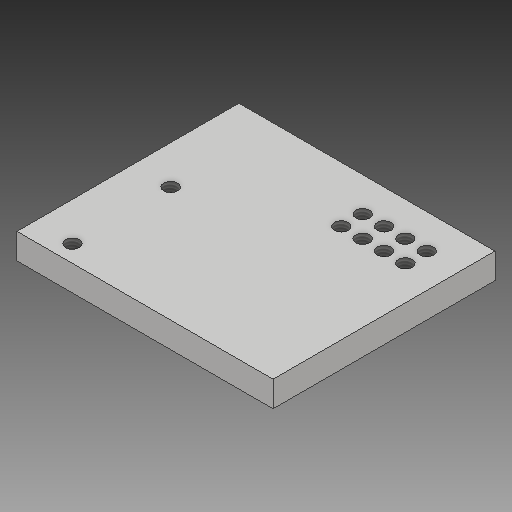
# Autodesk Inventor part: 160624 base pequeña laser
Saved by Autodesk Inventor 2019.2 (Build 232265000, 265)
## iProperties
Created: 2016-06-28
Part Number: 160624 base pequeña laser
Material: Generic
Document SubType Name: Modeling
Designer: Luis Villegas
Density: 1 g/cm^3
Appearance: Default
Author: Luis Villegas
Autodesk Inventor part; units mm, degrees
ref_plane "YZ Plane" through (0, 0, 0) normal (1, 0, 0) x (0, 1, 0)
ref_plane "XZ Plane" through (0, 0, 0) normal (0, 1, 0) x (-1, 0, 0)
ref_plane "XY Plane" through (0, 0, 0) normal (0, 0, 1) x (1, 0, 0)
sketch "Sketch1" plane through (0, 0, 0) normal (0, 1, 0) x (-1, 0, 0)
  line L0 (0, 0) -> (-52, 0)
  line L1 (-52, 0) -> (-52, -60)
  line L2 (-52, -60) -> (0, -60)
  line L3 (0, -60) -> (0, 0)
  dimension "d0" = 52
  dimension "d1" = 60
  constraints: 8 end point, 2 parallel, 1 coincident, 1 horizontal, 1 perpendicular
  measures "d0" distance of L2.end L1.end
  measures "d1" distance of L1.end L0.end
extrude "Extrusion1" add sketch "Sketch1" against normal blind 6
sketch "Sketch2" plane through (0, 0, 0) normal (0, 1, 0) x (1, 0, 0)
  line L0 (0, 0) -> (52, 0) projected
  line L1 (52, 0) -> (52, 60) projected
  point P0 (13, 37)
  point P1 (13, 42)
  point P2 (13, 47)
  point P3 (13, 52)
  point P4 (8, 37)
  point P5 (8, 42)
  point P6 (8, 47)
  point P7 (8, 52)
  point P8 (48, 9)
  point P9 (25, 9)
  dimension "d12" = 39
  dimension "d13" = 37
  dimension "d14" = 42
  dimension "d15" = 47
  dimension "d16" = 52
  dimension "d17" = 5
  dimension "d31" = 4
  dimension "d32" = 9
  dimension "d33" = 27
  dimension "d34" = 9
  constraints: 6 vertical alignment, 4 horizontal alignment
  measures "d12" distance from line of L1 point (13, 37)
  measures "d13" distance from line of L0 point (13, 37)
  measures "d14" distance from line of L0 point (13, 42)
  measures "d15" distance from line of L0 point (13, 47)
  measures "d16" distance from line of L0 point (13, 52)
  measures "d17" distance of point (13, 37) point (8, 37)
  measures "d31" distance from line of L1 point (48, 9)
  measures "d32" distance from line of L0 point (48, 9)
  measures "d33" distance from line of L1 point (25, 9)
  measures "d34" distance from line of L0 point (25, 9)
hole "Hole3" at (13, 0, -37) at (13, 0, -42) at (13, 0, -47) at (13, 0, -52) at (8, 0, -37) at (8, 0, -42) at (8, 0, -47) at (8, 0, -52) at (48, 0, -9) at (25, 0, -9) direction (0, -1, 0) diameter 3.242 end through all thread size "M4x0.7" class "6H" standard "ANSI Metric M Profile"
body "Solid1"
